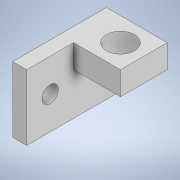
# Autodesk Inventor part: IRSensorMount
Saved by Autodesk Inventor 2020.3 (Build 243373000, 373)
## iProperties
Created: 2020-08-18
Part Number: IRSensorMount
Material: Generic
Document SubType Name: Modeling
Designer: joesp
Density: 1 g/cm^3
Appearance: Default
Author: joesp
Autodesk Inventor part; units mm, degrees
ref_plane "YZ Plane" through (0, 0, 0) normal (1, 0, 0) x (0, 1, 0)
ref_plane "XZ Plane" through (0, 0, 0) normal (0, 1, 0) x (-1, 0, 0)
ref_plane "XY Plane" through (0, 0, 0) normal (0, 0, 1) x (1, 0, 0)
sketch "Sketch2" plane through (0, 0, 0) normal (1, 0, 0) x (0, 1, 0)
  line L0 (0, 0) -> (14, 0)
  circle A0 centre (7, -5) radius 1.75
  line L1 (14, 0) -> (14, -20)
  line L2 (14, -20) -> (0, -20)
  line L3 (0, -20) -> (0, 0)
  point P0 (7, -20)
  dimension "d6" = 14
  dimension "d7" = 3.5
  dimension "d11" = 20
  dimension "d20" = 5
  constraints: 8 end point, 2 perpendicular, 1 centre point, 1 horizontal, 1 midpoint, 1 vertical, 1 vertical alignment
  measures "d6" distance of L0.start L0.end
  measures "d7" diameter of A0
  measures "d11" distance of L0.end L1.end
  measures "d20" distance from line of L0 A0.centre
extrude "Extrusion1" add sketch "Sketch2" along normal blind 3
sketch "Sketch3" plane through (3, 0, 0) normal (1, 0, 0) x (0, 0, -1)
  line L0 (20, 14) -> (10, 14)
  line L1 (10, 14) -> (10, 9)
  line L2 (10, 9) -> (20, 9)
  line L3 (20, 9) -> (20, 14)
  line L4 (20, 0) -> (20, 14) projected
  dimension "d12" = 5
  dimension "d13" = 10
  constraints: 8 end point, 2 perpendicular, 2 point on line, 1 parallel
  measures "d12" distance of L0.end L1.end
  measures "d13" distance of L1.end L2.end
extrude "Extrusion2" add sketch "Sketch3" along normal blind 10
sketch "Sketch4" plane through (3, 9, -10) normal (0, -1, 0) x (1, 0, 0)
  circle A0 centre (5, -5) radius 3
  line L0 (10, 0) -> (10, -10) projected
  point P0 (-3, 10)
  point P1 (10, -5)
  dimension "d16" = 6
  dimension "d17" = 5
  constraints: 1 centre point, 1 horizontal alignment, 1 midpoint
  measures "d16" diameter of A0
  measures "d17" distance from line of L0 A0.centre
extrude "Extrusion3" cut sketch "Sketch4" against normal through all
body "Solid1"
